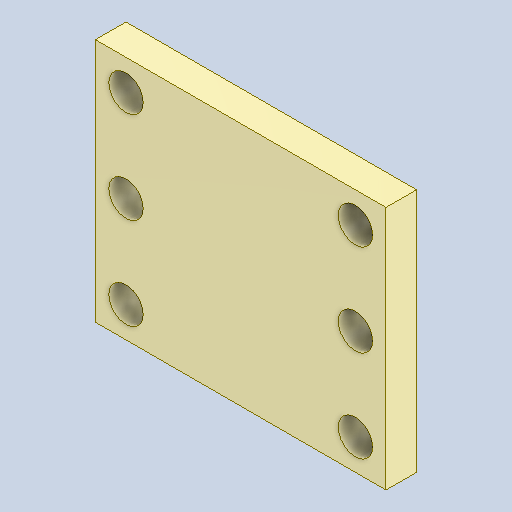
# Autodesk Inventor part: RD004_スペーサ
Saved by Autodesk Inventor 2022 (Build 260153000, 153)
## iProperties
Created: 2021-10-14
Part Number: RD004_スペーサ
Material: ナイロン 6/6
Document SubType Name: Modeling
Designer: gilte
Density: 1.13 g/cm^3
Appearance: ナイロン 6
Author: gilte
Autodesk Inventor part; units mm, degrees
ref_plane "YZ Plane" through (0, 0, 0) normal (1, 0, 0) x (0, 1, 0)
ref_plane "XZ Plane" through (0, 0, 0) normal (0, 1, 0) x (-1, 0, 0)
ref_plane "XY Plane" through (0, 0, 0) normal (0, 0, 1) x (1, 0, 0)
sketch "スケッチ1" plane through (0, 0, 0) normal (0, 0, 1) x (1, 0, 0)
  line L0 (0, 0) -> (38, 0)
  line L1 (38, 0) -> (38, 32)
  line L2 (38, 32) -> (0, 32)
  line L3 (0, 32) -> (0, 0)
  dimension "d0" = 38
  dimension "d1" = 32
  constraints: 8 end point, 2 parallel, 1 horizontal, 1 perpendicular
  measures "d0" distance of L2.end L1.end
  measures "d1" distance of L1.end L0.end
extrude "押し出し1" add sketch "スケッチ1" along normal blind 4
sketch "スケッチ2" plane through (0, 0, 4) normal (0, 0, 1) x (1, 0, 0)
  line L0 (0, 0) -> (38, 0) projected
  line L1 (0, 32) -> (0, 0) projected
  point P0 (4, 4)
  point P1 (4, 28)
  point P2 (34, 4)
  point P3 (34, 28)
  dimension "d4" = 4
  dimension "d5" = 4
  dimension "d8" = 24
  dimension "d11" = 30
  constraints: 1 horizontal, 1 vertical, 3 other
  measures "d4" distance from line of L0 point (4, 4)
  measures "d5" distance from line of L1 point (4, 4)
  measures "d8" distance of point (4, 4) point (4, 28)
  measures "d11" distance of point (4, 4) point (34, 4)
hole "穴1" at (4, 4, 4) at (4, 28, 4) at (34, 4, 4) at (34, 28, 4) direction (0, 0, -1) diameter 4.5 end through all
sketch "スケッチ3" plane through (0, 0, 4) normal (0, 0, 1) x (1, 0, 0)
  line L0 (0, 32) -> (0, 0) projected
  line L1 (0, 16) -> (4, 16)
  line L2 (34, 16) -> (38, 16)
  line L3 (38, 0) -> (38, 32) projected
  line L4 (4, 16) -> (34, 16)
  dimension "d28" = 30
  constraints: 6 end point, 2 coincident, 2 horizontal, 2 midpoint, 1 collinear
  measures "d28" distance of L4.start L4.end
hole "穴2" at (4, 16, 4) at (34, 16, 4) direction (0, 0, -1) diameter 4.5 depth 4 clearance for "Countersunk Flat Head Screw ISO 2009/7046" size "M4" standard "ISO"
